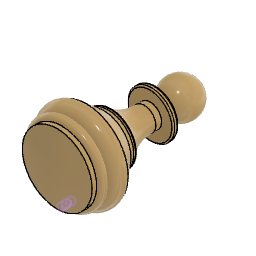
P3 (Autodesk Fusion 360 design; units mm, degrees)
Autodesk Fusion 360 part; units mm, degrees
sketch "Sketch1" plane through (0, 0, 0) normal (0, 1, 0) x (1, 0, 0)
  circle A0 centre (0, 0) radius 7.5
  dimension "d1" = 15
  constraint coincident A0.centre origin
  measures "d1" diameter of A0
extrude "Extrude1" add sketch "Sketch1" along normal blind 1
sketch "Sketch2" plane through (0, 0, 0) normal (1, 0, 0) x (0, 1, 0)
  line L0 (1, 0) -> (1.1751, 0)
  line L1 (1.1751, 0) -> (3, 0)
  line L2 (3, 0) -> (3, -7.5)
  arc A0 (1, -7.5) -> (3, -7.5) centre (2, -7.5) ccw
  line L3 (1, 0) -> (1, -0.3)
  line L4 (1, -0.3) -> (1, -7.5)
  constraint horizontal L0
  constraint parallel L0 L1
  constraint perpendicular L1 L2
  constraint tangent L2 A0
  constraint perpendicular L0 L3
  constraint tangent A0 L4
  constraint vertical L4
sketch "Sketch3" plane through (0, 0, 0) normal (1, 0, 0) x (0, 1, 0)
  arc A0 (1, -7.5) -> (3, -7.5) centre (2, -7.5) ccw
  dimension "d4" = 1
  measures "d4" radius of A0
revolve "Revolve1" add sketch "Sketch2" angle 360 about axis through (0, 1.1751, 0) along (0, 1, 0)
sketch "Sketch4" plane through (0, 0, 0) normal (1, 0, 0) x (0, 1, 0)
  line L0 (3, 0) -> (11.5, 0)
  line L1 (11.5, 0) -> (11.5, -5.5)
  line L2 (11.5, -5.5) -> (11, -5.5)
  arc A0 (11, -5.5) -> (10.0358, -5.8509) centre (11, -7) ccw
  line L3 (10.0358, -5.8509) -> (6.2853, -8.998)
  arc A1 (3, -7.5) -> (6.2853, -8.998) centre (4.9997, -7.4659) ccw
  line L4 (3, 0) -> (3, -7.5)
  point P0 (3, -7.5)
  dimension "d6" = 40
  dimension "d7" = 7
  dimension "d8" = 1.5
  dimension "d9" = 11.5
  dimension "d10" = 0.5
  dimension "d11" = 2
  dimension "d12" = 3
  constraint perpendicular L0 L1
  constraint tangent L2 A0
  constraint tangent A0 L3
  constraint tangent L3 A1
  constraint vertical L1
  constraint horizontal L0.start origin
  constraint vertical L0.start P0
  constraint coincident P0 A1.start
  constraint horizontal L2
  measures "d6" angle of L0 L3
  measures "d7" vertical distance of L0.end A0.centre
  measures "d8" radius of A0
  measures "d9" horizontal distance of L0.end origin
  measures "d10" horizontal distance of L1.end A0.centre
  measures "d11" radius of A1
  measures "d12" distance of origin L0.start
revolve "Revolve2" add sketch "Sketch4" angle 360 about axis through (0, 3, 0) along (0, 1, 0)
sketch "Sketch5" plane through (0, 0, 0) normal (1, 0, 0) x (0, 1, 0)
  line L0 (11.5, 0) -> (11.5, -5.5)
  line L1 (11.5, 0) -> (20, 0)
  line L2 (20, 0) -> (20, -2.5)
  line L3 (20, -2.5) -> (18.75, -2.5)
  arc A0 (18.75, -2.5) -> (11.5, -5.5) centre (18.642, -12.4994) ccw
  point P0 (11.5, -5.5)
  dimension "d14" = 5.5
  dimension "d15" = 2.5
  dimension "d16" = 20
  dimension "d17" = 1.25
  dimension "d18" = 10
  constraint vertical L0
  constraint perpendicular L0 L1
  constraint perpendicular L1 L2
  constraint perpendicular L2 L3
  constraint coincident P0 L0.end
  measures "d14" distance of P0 L1
  measures "d15" distance of L1.end L2.end
  measures "d16" distance of origin L2
  measures "d17" distance of L2.end L3.end
  measures "d18" radius of A0
revolve "Revolve3" add sketch "Sketch5" angle 360 about axis through (0, 11.5, 0) along (0, 1, 0)
sketch "Sketch6" plane through (0, 0, 0) normal (1, 0, 0) x (0, 1, 0)
  line L0 (20, 0) -> (23, 0)
  line L1 (20, 0) -> (20, -5)
  line L2 (20, -5) -> (21, -5)
  arc A0 (21, -5) -> (23, 0) centre (13.0581, 1.0767) ccw
  line L3 (20, 2.5) -> (20, -2.5)
  point P0 (20, 0)
  point P1 (20, 0)
  dimension "d20" = 3
  dimension "d21" = 5
  dimension "d22" = 1
  dimension "d23" = 10
  constraint horizontal L0
  constraint perpendicular L0 L1
  constraint perpendicular L1 L2
  constraint coincident P0 L0.start
  constraint coincident P1 L3
  constraint midpoint L3 P1
  constraint coincident P1 P0
  measures "d20" distance of P0 L0.end
  measures "d21" distance of P0 L1.end
  measures "d22" distance of L1.end L2.end
  measures "d23" radius of A0
revolve "Revolve4" add sketch "Sketch6" angle 360 about axis through (0, 20, 0) along (0, 1, 0)
sketch "Sketch7" plane through (0, 0, 0) normal (1, 0, 0) x (0, 1, 0)
  line L0 (22.5, 0) -> (30.5, 0)
  arc A0 (22.5, 0) -> (30.5, 0) centre (26.5, 0) ccw
  dimension "d25" = 26.5
  dimension "d26" = 8
  constraint horizontal L0
  measures "d25" distance of origin A0.centre
  measures "d26" diameter of A0
revolve "Revolve5" add sketch "Sketch7" angle 360 about axis through (0, 22.5, 0) along (0, 1, 0)
fillet "Fillet1" radius 0.3 3 edges at (-4.6616, 21, -1.8081) (-4.6616, 20, -1.8081) (-5.1278, 11.5, -1.9889)
